Autodesk Fusion 360 part; units mm, degrees
(part 2 of 2)
sketch "top shell" plane through (0, 0, 8) normal (0, 0, 1) x (1, 0, 0) in component "diag_up_top"
  line L0 (2.8575, 28.7338) -> (4.2862, 28.7338) construction
  line L1 (1.4287, 28.7338) -> (2.8575, 28.7338) construction
  line L2 (1.4287, 8.4138) -> (1.4287, 28.7338) construction
  line L3 (4.2862, 28.7338) -> (10.6363, 28.7338) construction
  line L4 (10.6363, 28.7338) -> (10.6363, 20.6376) construction
  line L5 (10.6363, 20.6376) -> (10.6363, 16.5099) construction
  line L6 (10.6363, 16.5099) -> (10.6363, 8.4138) construction
  line L7 (10.6363, 8.4138) -> (4.2862, 8.4138) construction
  line L8 (4.2862, 8.4138) -> (2.8575, 8.4138) construction
  line L9 (2.8575, 8.4138) -> (1.4287, 8.4138) construction
  line L10 (16.84, 48.2537) -> (16.84, 54.6038) construction
  line L11 (16.84, 54.6038) -> (24.9362, 54.6038) construction
  line L12 (16.84, 46.825) -> (16.84, 48.2537) construction
  line L13 (16.84, 45.3962) -> (16.84, 46.825) construction
  line L14 (37.16, 45.3962) -> (16.84, 45.3962) construction
  line L15 (37.16, 46.825) -> (37.16, 45.3962) construction
  line L16 (37.16, 48.2537) -> (37.16, 46.825) construction
  line L17 (37.16, 54.6038) -> (37.16, 48.2537) construction
  line L18 (29.0638, 54.6038) -> (37.16, 54.6038) construction
  line L19 (24.9362, 54.6038) -> (29.0638, 54.6038) construction
  line L20 (46.2537, 45.16) -> (52.6038, 45.16) construction
  line L21 (44.825, 45.16) -> (46.2537, 45.16) construction
  line L22 (43.3962, 45.16) -> (44.825, 45.16) construction
  line L23 (43.3962, 24.84) -> (43.3962, 45.16) construction
  line L24 (52.6038, 45.16) -> (52.6038, 37.0638) construction
  line L25 (52.6038, 37.0638) -> (52.6038, 32.9362) construction
  line L26 (52.6038, 32.9362) -> (52.6038, 24.84) construction
  line L27 (52.6038, 24.84) -> (46.2537, 24.84) construction
  line L28 (46.2537, 24.84) -> (44.825, 24.84) construction
  line L29 (44.825, 24.84) -> (43.3962, 24.84) construction
  line L30 (43.3962, 23.62) -> (44.825, 23.62) construction
  line L31 (44.825, 23.62) -> (46.2537, 23.62) construction
  line L32 (46.2537, 23.62) -> (52.6038, 23.62) construction
  line L33 (52.6038, 23.62) -> (52.6038, 17.27) construction
  line L34 (43.3962, 8.38) -> (43.3962, 23.62) construction
  line L35 (44.825, 8.38) -> (43.3962, 8.38) construction
  line L36 (46.2537, 8.38) -> (44.825, 8.38) construction
  line L37 (52.6038, 8.38) -> (46.2537, 8.38) construction
  line L38 (52.6038, 14.73) -> (52.6038, 8.38) construction
  line L39 (52.6038, 17.27) -> (52.6038, 14.73) construction
  circle A0 centre (49, 51) radius 1.5875 construction
  circle A1 centre (57.25, 6.25) radius 1.75 construction
  circle A2 centre (-4.25, 6.25) radius 1.75 construction
  circle A3 centre (4, 51) radius 1.5875 construction
  line L40 (0, 1) -> (0, 54) construction
  line L41 (53, 1) -> (53, 54) construction
  line L42 (60.5, 2) -> (-7.5, 2)
  line L43 (60.5, 0) -> (-7.5, 0)
  arc A4 (-10.5, 3) -> (-7.5, 0) centre (-7.5, 3) ccw
  arc A5 (-8.5, 3) -> (-7.5, 2) centre (-7.5, 3) ccw
  line L44 (-8.5, 3) -> (-8.5, 54.5)
  line L45 (-10.5, 3) -> (-10.5, 54.5)
  arc A6 (-7.5, 55.5) -> (-8.5, 54.5) centre (-7.5, 54.5) ccw
  arc A7 (-7.5, 57.5) -> (-10.5, 54.5) centre (-7.5, 54.5) ccw
  line L46 (-7.5, 57.5) -> (60.5, 57.5)
  line L47 (-7.5, 55.5) -> (60.5, 55.5)
  arc A8 (63.5, 54.5) -> (60.5, 57.5) centre (60.5, 54.5) ccw
  arc A9 (61.5, 54.5) -> (60.5, 55.5) centre (60.5, 54.5) ccw
  line L48 (63.5, 54.5) -> (63.5, 3)
  line L49 (61.5, 54.5) -> (61.5, 3)
  arc A10 (60.5, 0) -> (63.5, 3) centre (60.5, 3) ccw
  arc A11 (60.5, 2) -> (61.5, 3) centre (60.5, 3) ccw
  line L50 (0, 2) -> (0, 0)
  line L51 (53, 2) -> (53, 0)
  arc A12 (62.7, 54.5) -> (60.5, 56.7) centre (60.5, 54.5) ccw
  line L52 (-7.5, 56.7) -> (60.5, 56.7)
  arc A13 (-7.5, 56.7) -> (-9.7, 54.5) centre (-7.5, 54.5) ccw
  line L53 (-9.7, 3) -> (-9.7, 54.5)
  arc A14 (-9.7, 3) -> (-7.5, 0.8) centre (-7.5, 3) ccw
  arc A15 (60.5, 0.8) -> (62.7, 3) centre (60.5, 3) ccw
  line L54 (62.7, 54.5) -> (62.7, 3)
  line L55 (60.5, 0.8) -> (53, 0.8)
  line L56 (0, 0.8) -> (-7.5, 0.8)
  circle A16 centre (4, 51) radius 1.25
  circle A17 centre (57.25, 6.25) radius 1.25
  circle A18 centre (-4.25, 6.25) radius 1.25
  circle A19 centre (49, 51) radius 1.25
  circle A20 centre (4, 51) radius 3
  circle A21 centre (49, 51) radius 3
  circle A22 centre (57.25, 6.25) radius 3
  circle A23 centre (-4.25, 6.25) radius 3
  line L57 (16.74, 44.7962) -> (37.26, 44.7962)
  line L58 (37.76, 45.2962) -> (37.76, 54.7038)
  line L59 (37.26, 55.2038) -> (16.74, 55.2038)
  line L60 (16.24, 54.7038) -> (16.24, 45.2962)
  line L61 (10.7363, 7.8138) -> (1.3287, 7.8138)
  line L62 (0.8287, 8.3138) -> (0.8287, 28.8338)
  line L63 (1.3287, 29.3338) -> (10.7363, 29.3338)
  line L64 (11.2363, 28.8338) -> (11.2363, 8.3138)
  line L65 (43.2962, 7.78) -> (52.7038, 7.78)
  line L66 (53.2038, 8.28) -> (53.2038, 45.26)
  line L67 (52.7038, 45.76) -> (43.2962, 45.76)
  line L68 (42.7962, 45.26) -> (42.7962, 8.28)
  arc A24 (1.3287, 29.3338) -> (0.8287, 28.8338) centre (1.3287, 28.8338) ccw
  arc A25 (11.2363, 28.8338) -> (10.7363, 29.3338) centre (10.7363, 28.8338) ccw
  arc A26 (10.7363, 7.8138) -> (11.2363, 8.3138) centre (10.7363, 8.3138) ccw
  arc A27 (0.8287, 8.3138) -> (1.3287, 7.8138) centre (1.3287, 8.3138) ccw
  arc A28 (16.74, 55.2038) -> (16.24, 54.7038) centre (16.74, 54.7038) ccw
  arc A29 (16.24, 45.2962) -> (16.74, 44.7962) centre (16.74, 45.2962) ccw
  arc A30 (37.26, 44.7962) -> (37.76, 45.2962) centre (37.26, 45.2962) ccw
  arc A31 (37.76, 54.7038) -> (37.26, 55.2038) centre (37.26, 54.7038) ccw
  arc A32 (43.2962, 45.76) -> (42.7962, 45.26) centre (43.2962, 45.26) ccw
  arc A33 (53.2038, 45.26) -> (52.7038, 45.76) centre (52.7038, 45.26) ccw
  arc A34 (52.7038, 7.78) -> (53.2038, 8.28) centre (52.7038, 8.28) ccw
  arc A35 (42.7962, 8.28) -> (43.2962, 7.78) centre (43.2962, 8.28) ccw
  dimension "d100" = 0.8
  dimension "d101" = 2.5
  dimension "d102" = 2.5
  dimension "d103" = 2.5
  dimension "d104" = 2.5
  dimension "d105" = 6
  dimension "d106" = 6
  dimension "d107" = 6
  dimension "d108" = 6
  dimension "d109" = 0.6
  dimension "d110" = 0.6
  dimension "d111" = 0.6
  dimension "d112" = 0.6
  dimension "d113" = 0.6
  dimension "d114" = 0.6
  dimension "d115" = 0.6
  dimension "d116" = 0.6
  dimension "d117" = 0.6
  dimension "d118" = 0.6
  dimension "d119" = 0.6
  dimension "d120" = 0.6
  dimension "d121" = 0.5
  dimension "d122" = 0.5
  dimension "d123" = 0.5
  constraint coincident L42 L50.start
  constraint coincident L40 L50.start
  constraint coincident L50.end origin
  constraint coincident L42 L51.start
  constraint coincident L41 L51.start
  constraint coincident L43 L51.end
  constraint perpendicular L43 L51
  constraint concentric A8 A12
  constraint parallel L46 L52
  constraint concentric A7 A13
  constraint parallel L45 L53
  constraint concentric A4 A14
  constraint parallel L43 L55
  constraint concentric A10 A15
  constraint parallel L48 L54
  constraint tangent A15 L54
  constraint tangent L53 A14
  constraint tangent A12 L54
  constraint tangent A12 L52
  constraint tangent L52 A13
  constraint tangent A13 L53
  constraint tangent A15 L55
  constraint tangent A14 L55
  constraint coincident L51 L55.end
  constraint coincident L50 L56.start
  constraint collinear L55 L56
  constraint concentric A3 A16
  constraint concentric A1 A17
  constraint concentric A2 A18
  constraint concentric A0 A19
  constraint concentric A16 A20
  constraint concentric A19 A21
  constraint concentric A17 A22
  constraint concentric A18 A23
  constraint horizontal L57
  constraint vertical L58
  constraint horizontal L59
  constraint vertical L60
  constraint horizontal L61
  constraint vertical L62
  constraint horizontal L63
  constraint vertical L64
  constraint horizontal L65
  constraint vertical L66
  constraint horizontal L67
  constraint vertical L68
  constraint tangent L62 A24
  constraint tangent L63 A24
  constraint tangent L63 A25
  constraint tangent L64 A25
  constraint equal A24 A25
  constraint tangent L61 A26
  constraint tangent L64 A26
  constraint equal A24 A26
  constraint tangent L61 A27
  constraint tangent L62 A27
  constraint equal A24 A27
  constraint tangent L59 A28
  constraint tangent L60 A28
  constraint tangent L57 A29
  constraint tangent L60 A29
  constraint equal A28 A29
  constraint tangent L57 A30
  constraint tangent L58 A30
  constraint equal A28 A30
  constraint tangent L58 A31
  constraint tangent L59 A31
  constraint equal A28 A31
  constraint tangent L67 A32
  constraint tangent L68 A32
  constraint tangent L66 A33
  constraint tangent L67 A33
  constraint equal A32 A33
  constraint tangent L65 A34
  constraint tangent L66 A34
  constraint equal A32 A34
  constraint tangent L65 A35
  constraint tangent L68 A35
  constraint equal A32 A35
  measures "d100" distance of L46 L52
  measures "d101" diameter of A16
  measures "d102" diameter of A17
  measures "d103" diameter of A18
  measures "d104" diameter of A19
  measures "d105" diameter of A20
  measures "d106" diameter of A21
  measures "d107" diameter of A22
  measures "d108" diameter of A23
  measures "d109" distance of L11 L59
  measures "d110" distance of L14 L57
  measures "d111" distance of L13 L60
  measures "d112" distance of L15 L58
  measures "d113" distance of L22 L67
  measures "d114" distance of L23 L68
  measures "d115" distance of L24 L66
  measures "d116" distance of L37 L65
  measures "d117" distance of L3 L63
  measures "d118" distance of L4 L64
  measures "d119" distance of L2 L62
  measures "d120" distance of L7 L61
  measures "d121" radius of A24
  measures "d122" radius of A28
  measures "d123" radius of A32
extrude "Extrude1''" add sketch "top shell" along normal blind 2 separate body contours L42 A5 L44 A6 L47 A9 L49 A11 L50 L51 A12 L52 A13 L53 A14 A15 L54 L55 L56 | L42 A5 L44 A6 L47 A9 L49 A11 | L42 L43 L50 L51 | L43 A4 L45 A7 L46 A8 L48 A10 L50 L51 A12 L52 A13 L53 A14 A15 L54 L55 L56 | A16 | A17 | A18 | A19 | A20 | A21 | A22 | A23 makes body 3 in component "diag_up_top"
extrude "Extrude2''" add sketch "top shell" against normal blind 7.8 contours A20 | A21 bodies 3 in component "diag_up_top"
extrude "Extrude3''" add sketch "top shell" against normal blind 7.8 contours A22 | A23 bodies 3 in component "diag_up_top"
extrude "Extrude4''" add sketch "top shell" against normal blind 2.5 contours L42 A5 L44 A6 L47 A9 L49 A11 L50 L51 A12 L52 A13 L53 A14 A15 L54 L55 L56 bodies 3 in component "diag_up_top"
extrude "Extrude5''" add sketch "top shell" against normal blind 3.5 contours L43 A4 L45 A7 L46 A8 L48 A10 L50 L51 A12 L52 A13 L53 A14 A15 L54 L55 L56 bodies 3 in component "diag_up_top"
extrude "Extrude6''" add sketch "top shell" against normal blind 5 contours L42 L43 L50 L51 bodies 3 in component "diag_up_top"
fillet "Fillet1'" radius 1 8 edges at (63.5, 28.75, 10) (62.6213, 56.6213, 10) (26.5, 57.5, 10) (-9.6213, 56.6213, 10) (-10.5, 28.75, 10) (-9.6213, 0.8787, 10) (26.5, 0, 10) (62.6213, 0.8787, 10) on bodies 3 in component "diag_up_top"
fillet "Fillet4'" radius 0.5 4 edges at (-7.047, 5.1652, 8) (1.203, 49.9152, 8) (46.203, 49.9152, 8) (54.453, 5.1652, 8) on bodies 3 in component "diag_up_top"
fillet "Fillet5'" radius 0.5 8 edges at (-8.5, 28.75, 8) (-8.2071, 55.2071, 8) (26.5, 55.5, 8) (61.2071, 55.2071, 8) (61.5, 28.75, 8) (61.2071, 2.2929, 8) (26.5, 2, 8) (-8.2071, 2.2929, 8) on bodies 3 in component "diag_up_top"
component "PCB" placed x (1, 0, 0) y (0, 1, 0) z (0, 0, 1) at (0, 0, 0)
component "diag_up_bottom" placed x (1, 0, 0) y (0, 1, 0) z (0, 0, 1) at (0, 0, 0)
component "diag_up_top" placed x (1, 0, 0) y (0, 1, 0) z (0, 0, 1) at (0, 0, 0)
equation "pcb_thickness = 1.6 mm"
equation "below = 2.8 mm + pcb_thickness"
equation "wall = 2 mm"
equation "width = 70 mm + 2 * wall"
equation "length = pcb_length + 0.5 mm + wall"
equation "above = 10 mm - wall"
equation "pcb_width = 53 mm"
equation "pcb_length = 55 mm"
equation "r_corner = 3 mm"
equation "drill = 3.5 mm"
equation "d_screw = 6 mm"
equation "tol_x = 0.3 mm"
equation "tol_connector = 0.6 mm"
equation "d_post = 8.5 mm"
equation "d_post2 = 8 mm"
equation "bottom_height = 4.3 mm + below"
equation "overlap = 1 mm"
equation "top_height = above + below - bottom_height - tol_y"
equation "d34 = -below"
equation "d35 = tol_connector"
equation "d37 = d35"
equation "d47 = length"
equation "d48 = r_corner"
equation "d49 = ( width - pcb_width ) / 2"
equation "d50 = width"
equation "d51 = wall"
equation "d53 = drill"
equation "d54 = d_screw"
equation "d56 = drill"
equation "d57 = d_screw"
equation "d58 = d_post"
equation "d59 = ( width - pcb_width - 2 * wall ) / 4"
equation "d60 = d59"
equation "d61 = drill"
equation "d64 = tol_x"
equation "d65 = tol_x"
equation "d66 = drill"
equation "d67 = d59"
equation "d68 = d67"
equation "d71 = d_post"
equation "d72 = wall * 0.6"
equation "d73 = -wall"
equation "d77 = bottom_height + overlap"
equation "d79 = bottom_height"
equation "d81 = below - pcb_thickness"
equation "d83 = below"
equation "d88 = tol_x"
equation "d89 = d86"
equation "d90 = d87"
equation "d91 = tol_x"
equation "d98 = above"
equation "d100 = wall * 0.4"
equation "d105 = d_screw"
equation "d106 = d_screw"
equation "d107 = d_screw"
equation "d108 = d_screw"
equation "d109 = tol_connector"
equation "d110 = tol_connector"
equation "d111 = tol_connector"
equation "d112 = tol_connector"
equation "d113 = tol_connector"
equation "d114 = tol_connector"
equation "d115 = tol_connector"
equation "d116 = tol_connector"
equation "d117 = tol_connector"
equation "d118 = tol_connector"
equation "d119 = tol_connector"
equation "d120 = tol_connector"
equation "d124 = wall"
equation "d126 = -above + tol_y"
equation "d128 = -above + tol_y"
equation "d130 = -top_height + overlap"
equation "d132 = -top_height"
equation "d138 = -top_height - 1.5 mm"
equation "tol_y = 0.2 mm"
named bodies: "PCB", "top shell"
